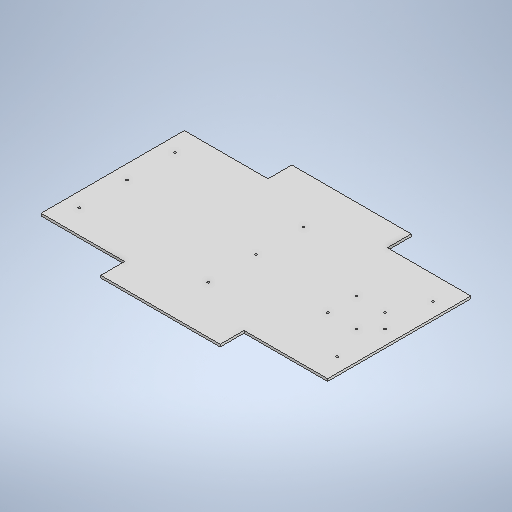
# Autodesk Inventor part: вверхняя плита
Saved by Autodesk Inventor 2025 (Build 290162000, 162)
## iProperties
Created: 2025-02-24
Part Number: вверхняя плита
Material: Типовые
Document SubType Name: Modeling
Designer: volko
Density: 1 g/cm^3
Appearance: По умолчанию
Author: volko
Autodesk Inventor part; units mm, degrees
ref_plane "YZ Plane" through (0, 0, 0) normal (1, 0, 0) x (0, 1, 0)
ref_plane "XZ Plane" through (0, 0, 0) normal (0, 1, 0) x (-1, 0, 0)
ref_plane "XY Plane" through (0, 0, 0) normal (0, 0, 1) x (1, 0, 0)
sketch "Эскиз1" plane through (0, 0, 0) normal (0, 1, 0) x (-1, 0, 0)
  line L0 (-300, 150) -> (-300, -150)
  line L1 (300, -150) -> (300, 150)
  line L2 (0, -280) -> (0, 280) projected
  line L3 (420, 0) -> (-420, 0) projected
  line L4 (125, 150) -> (125, 200)
  line L5 (125, 200) -> (-125, 200)
  line L6 (-125, 200) -> (-125, 150)
  line L7 (300, 150) -> (125, 150)
  line L8 (-125, 150) -> (-300, 150)
  line L9 (125, -150) -> (125, -200)
  line L10 (125, -200) -> (-125, -200)
  line L11 (-125, -200) -> (-125, -150)
  line L12 (-300, -150) -> (-125, -150)
  line L13 (125, -150) -> (300, -150)
  point P0 (0, 0)
  dimension "d0" = 600
  dimension "d1" = 300
  dimension "d39" = 400
  dimension "d40" = 250
  constraints: 24 end point, 5 parallel, 4 perpendicular, 4 symmetric about line, 2 horizontal, 1 collinear, 1 vertical, 4 other
  measures "d0" distance of L1.end L0.start
  measures "d1" distance of L1.start L1.end
  measures "d39" distance between parallel lines of L10 L5
  measures "d40" distance of L4.end L5.end
extrude "Выдавливание1" add sketch "Эскиз1" along normal blind 5
sketch "Эскиз2" plane through (0, 5, 0) normal (0, 1, 0) x (1, 0, 0)
  line L0 (0, 280) -> (0, -280) projected
  line L1 (-420, 0) -> (420, 0) projected
  point P0 (0, 0)
  point P1 (240, 30)
  point P2 (0, 0)
  point P3 (270, 100)
  point P4 (180, 30)
  point P5 (240, -30)
  point P6 (180, -30)
  point P7 (0, 100)
  point P8 (270, 0)
  point P9 (0, 0)
  point P10 (270, -100)
  point P11 (0, -100)
  point P12 (-270, 100)
  point P13 (-270, 0)
  point P14 (-270, -100)
  dimension "d15" = 60
  dimension "d18" = 60
  dimension "d21" = 180
  dimension "d22" = 270
  dimension "d32" = 270
  dimension "d35" = 100
  constraints: 5 symmetric about line, 2 horizontal, 2 vertical, 1 coincident, 8 other
  measures "d15" distance of point (240, 30) point (180, 30)
  measures "d18" distance of point (240, 30) point (240, -30)
  measures "d21" distance from line of L0 point (180, 30)
  measures "d22" distance from line of point (270, 100) L0
  measures "d32" distance of point (270, 100) point (0, 100)
  measures "d35" distance of point (270, 100) point (270, 0)
hole "Отверстие1" at (0, 5, -100) at (0, 5, 100) at (0, 5, 0) at (180, 5, 30) at (180, 5, -30) at (240, 5, 30) at (240, 5, -30) at (270, 5, 100) at (270, 5, 0) at (270, 5, -100) at (-270, 5, 100) at (-270, 5, 0) at (-270, 5, -100) direction (0, -1, 0) diameter 4.5 end through all
